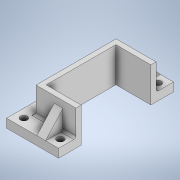
# Autodesk Inventor part: 2x1Attachment
Saved by Autodesk Inventor 2022 (Build 260153000, 153)
## iProperties
Created: 2022-02-14
Part Number: 2x1Attachment
Material: Generic
Document SubType Name: Modeling
Designer: Daniel Marquez
Density: 1 g/cm^3
Appearance: Default
Author: Daniel Marquez
Autodesk Inventor part; units mm, degrees
ref_plane "YZ Plane" through (0, 0, 0) normal (1, 0, 0) x (0, 1, 0)
sketch "Sketch1" plane through (0, 0, 0) normal (0, 1, 0) x (-1, 0, 0)
  line L0 (0, 0) -> (25.6032, 0) construction
  line L1 (25.6032, 0) -> (25.6032, -51) construction
  line L2 (25.6032, -51) -> (0, -51) construction
  line L3 (0, -51) -> (0, 0) construction
  line L4 (0, 0) -> (25.6032, 0)
  line L5 (33.02, 0) -> (33.02, 7.62)
  line L6 (33.02, 7.62) -> (0, 7.62)
  line L7 (0, 7.62) -> (0, 0)
  line L8 (0, -51) -> (25.6032, -51)
  line L9 (33.02, -51) -> (33.02, -58.62)
  line L10 (33.02, -58.62) -> (0, -58.62)
  line L11 (0, -58.62) -> (0, -51)
  line L12 (33.02, -58.62) -> (25.6032, -58.62)
  line L13 (25.6032, 7.62) -> (33.02, 7.62)
  line L14 (33.02, 7.62) -> (33.02, -58.62)
  line L15 (25.6032, 0) -> (25.6032, -51)
  line L16 (0, 0) -> (25.6032, 0)
  line L17 (29.21, 0) -> (29.21, 3.81)
  line L18 (29.21, 3.81) -> (0, 3.81)
  line L19 (0, 3.81) -> (0, 0)
  line L20 (0, -51) -> (25.6032, -51)
  line L21 (29.21, -51) -> (29.21, -54.81)
  line L22 (29.21, -54.81) -> (0, -54.81)
  line L23 (0, -54.81) -> (0, -51)
  line L24 (29.21, -54.81) -> (25.6032, -54.81)
  line L25 (25.6032, -51) -> (25.6032, 0)
  line L26 (25.6032, 3.81) -> (29.21, 3.81)
  line L27 (29.21, 3.81) -> (29.21, -54.81)
  line L28 (25.6032, 0) -> (25.6032, -51)
  dimension "d0" = 25.6032
  dimension "d1" = 51
  dimension "d2" = 33.02
  dimension "d3" = 7.62
  dimension "d4" = 33.02
  dimension "d5" = 7.62
  dimension "d6" = 29.21
  dimension "d7" = 3.81
  dimension "d8" = 29.21
  dimension "d9" = 3.81
  constraints: 58 end point, 13 parallel, 7 horizontal, 7 perpendicular, 2 point on line, 1 collinear
  measures "d0" distance of L1.end L2.end
  measures "d1" distance of L1.end L0.end
  measures "d2" distance of L6.end L5.end
  measures "d3" distance of L5.end L5.start
  measures "d4" distance of L9.end L10.end
  measures "d5" distance of L9.start L9.end
  measures "d6" distance of L18.end L17.end
  measures "d7" distance of L17.end L17.start
  measures "d8" distance of L21.end L22.end
  measures "d9" distance of L21.start L21.end
extrude "Extrusion1" add sketch "Sketch1" along normal blind 25.4 contours L7 L18 L17 L27 L21 L22 L11 L8 L15 L4
sketch "Sketch2" plane through (0, 0, 0) normal (0, -1, 0) x (1, 0, 0)
  line L0 (0, -51) -> (0, -54.81) projected
  line L1 (0, -54.81) -> (-29.21, -54.81)
  line L2 (-38.1, -54.81) -> (-38.1, -67.51)
  line L3 (-38.1, -67.51) -> (0, -67.51)
  line L4 (0, -67.51) -> (0, -54.81)
  line L5 (-29.21, 3.81) -> (0, 3.81) projected
  line L6 (0, 3.81) -> (-29.21, 3.81)
  line L7 (-38.1, 3.81) -> (-38.1, 16.51)
  line L8 (-38.1, 16.51) -> (0, 16.51)
  line L9 (0, 16.51) -> (0, 3.81)
  line L10 (-29.21, 3.81) -> (-29.21, -54.81)
  line L11 (-38.1, -54.81) -> (-38.1, 3.81)
  point P0 (0, 0)
  dimension "d14" = 38.1
  dimension "d15" = 12.7
  dimension "d16" = 38.1
  dimension "d17" = 12.7
  constraints: 20 end point, 5 parallel, 2 horizontal, 2 perpendicular
  measures "d14" distance of L3.end L2.end
  measures "d15" distance of L2.end L2.start
  measures "d16" distance of L7.end L8.end
  measures "d17" distance of L7.start L7.end
extrude "Extrusion3" add sketch "Sketch2" against normal blind 6.35
ref_plane "Work Plane1" through (-12.7, 0, 0) normal (1, 0, 0) x (0, 0, -1)
sketch "Sketch4" plane through (-12.7, 0, 0) normal (1, 0, 0) x (0, 0, -1)
  line L0 (-16.51, 6.35) -> (-3.81, 20.549)
  line L1 (67.51, 6.35) -> (54.81, 20.549)
  line L2 (67.51, 6.35) -> (-16.51, 6.35) projected
  line L3 (-16.51, 6.35) -> (-3.81, 6.35)
  line L4 (-3.81, 6.35) -> (-3.81, 25.4) projected
  line L5 (-3.81, 20.549) -> (-3.81, 6.35)
  line L6 (54.81, 6.35) -> (54.81, 25.4) projected
  line L7 (54.81, 20.549) -> (54.81, 6.35)
  line L8 (54.81, 6.35) -> (67.51, 6.35) projected
  line L9 (54.81, 6.35) -> (67.51, 6.35)
  point P0 (0, 0)
  dimension "d23" = 19.05
  dimension "d24" = 19.05
  constraints: 12 end point, 3 collinear, 1 point on line
  measures "d23" distance of L0.start L0.end
  measures "d24" distance of L1.start L1.end
extrude "Extrusion4" add sketch "Sketch4" along normal mid plane 6.35
ref_plane "Work Plane2" through (-29.21, 25.4, -25.4) normal (0, 0, 1) x (1, 0, 0)
sketch "Sketch5" plane through (-29.21, 25.4, -25.4) normal (0, 0, 1) x (1, 0, 0)
  line L0 (-8.89, -25.4) -> (-8.89, -19.05) projected
  line L1 (-8.89, -19.05) -> (0, -2.2015)
  line L2 (0, -19.05) -> (0, 0) projected
  line L3 (0, -2.2015) -> (0, -19.05)
  line L4 (13.335, -19.05) -> (-8.89, -19.05) projected
  line L5 (-8.89, -19.05) -> (0, -19.05)
  point P0 (29.21, -25.4)
  dimension "d28" = 19.05
  constraints: 6 end point, 1 collinear, 1 perpendicular, 1 point on line
  measures "d28" distance of L0.end L1.end
extrude "Extrusion5" add sketch "Sketch5" along normal mid plane 19.05
fillet "Fillet1" radius 1.5875 6 edges at (-29.21, 6.35, -6.0325) (-22.5425, 6.35, 3.81) (-4.7625, 6.35, 3.81) (-29.21, 6.35, -44.8675) (-22.5425, 6.35, -54.81) (-4.7625, 6.35, -54.81)
sketch "Sketch6" plane through (0, 6.35, 0) normal (0, 1, 0) x (1, 0, 0)
  circle A0 centre (-31.75, 61.16) radius 2.54
  circle A1 centre (-31.75, -10.16) radius 2.54
  line L0 (-15.875, 67.51) -> (-38.1, 67.51) projected
  line L1 (-38.1, 67.51) -> (-38.1, 34.925) projected
  line L2 (-38.1, -16.51) -> (-15.875, -16.51) projected
  line L3 (-38.1, 15.875) -> (-38.1, -16.51) projected
  circle A2 centre (-5.08, 61.16) radius 2.54
  circle A3 centre (-5.08, -10.16) radius 2.54
  line L4 (0, 67.51) -> (-9.525, 67.51) projected
  line L5 (0, 56.3975) -> (0, 67.51) projected
  line L6 (-9.525, -16.51) -> (0, -16.51) projected
  line L7 (0, -16.51) -> (0, -5.3975) projected
  point P0 (0, 0)
  dimension "d32" = 5.08
  dimension "d33" = 5.08
  dimension "d34" = 6.35
  dimension "d35" = 6.35
  dimension "d36" = 6.35
  dimension "d37" = 6.35
  dimension "d38" = 5.08
  dimension "d39" = 5.08
  dimension "d40" = 6.35
  dimension "d41" = 5.08
  dimension "d42" = 6.35
  dimension "d43" = 5.08
  constraints: 4 centre point
  measures "d32" diameter of A0
  measures "d33" diameter of A1
  measures "d34" distance from line of L0 A0.centre
  measures "d35" distance from line of L1 A0.centre
  measures "d36" distance from line of L2 A1.centre
  measures "d37" distance from line of L3 A1.centre
  measures "d38" diameter of A2
  measures "d39" diameter of A3
  measures "d40" distance from line of L4 A2.centre
  measures "d41" distance from line of L5 A2.centre
  measures "d42" distance from line of L6 A3.centre
  measures "d43" distance from line of L7 A3.centre
extrude "Extrusion6" cut sketch "Sketch6" against normal through all
body "Solid1"
